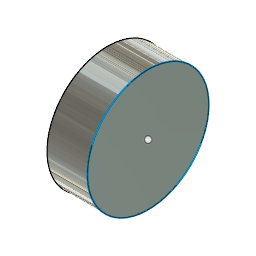
Iman (Autodesk Fusion 360 design; units mm, degrees)
Autodesk Fusion 360 part; units mm, degrees
sketch "sketch 290" plane through (6, 0, 0) normal (-1, 0, 0) x (0, -1, 0)
  circle A0 centre (-20, 44.4994) radius 3
extrude "Extruir1" add sketch "sketch 290" along normal blind 2
